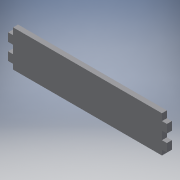
# Autodesk Inventor part: маленькое дно1
Saved by Autodesk Inventor 2019 (Build 230136000, 136)
## iProperties
Created: 2022-02-24
Part Number: маленькое дно1
Material: Типовые
Document SubType Name: Modeling
Designer: korsh
Density: 1 g/cm^3
Appearance: По умолчанию
Author: korsh
Autodesk Inventor part; units mm, degrees
ref_plane "YZ Plane" through (0, 0, 0) normal (1, 0, 0) x (0, 1, 0)
ref_plane "XZ Plane" through (0, 0, 0) normal (0, 1, 0) x (-1, 0, 0)
ref_plane "XY Plane" through (0, 0, 0) normal (0, 0, 1) x (1, 0, 0)
sketch "Эскиз1" plane through (0, 0, 0) normal (0, 0, 1) x (1, 0, 0)
  line L0 (0, 0) -> (0, -10) projected
  line L1 (0, 0) -> (-6, 0) projected
  line L2 (-6, -10) -> (-6, 0) projected
  line L3 (0, -10) -> (-6, -10) projected
  line L4 (0, -20) -> (0, -30) projected
  line L5 (0, -20) -> (-6, -20) projected
  line L6 (-6, -30) -> (-6, -20) projected
  line L7 (0, -30) -> (-6, -30) projected
  line L8 (0, -30) -> (0, -36.0265) projected
  line L9 (0, 8.1888) -> (0, 0) projected
  line L10 (186, -20) -> (186, -30) projected
  line L11 (186, -20) -> (180, -20) projected
  line L12 (180, -30) -> (180, -20) projected
  line L13 (186, -30) -> (180, -30) projected
  line L14 (186, 0) -> (186, -10) projected
  line L15 (186, 0) -> (180, 0) projected
  line L16 (180, -10) -> (180, 0) projected
  line L17 (186, -10) -> (180, -10) projected
  line L18 (180, -36.0265) -> (180, -30) projected
  line L19 (180, 0) -> (180, 8.1888) projected
  line L20 (0, 8.1888) -> (180, 8.1888)
  line L21 (180, 8.1888) -> (180, -36.0265)
  line L22 (180, -36.0265) -> (0, -36.0265)
  line L23 (0, -36.0265) -> (0, 8.1888)
  constraints: 8 end point, 2 parallel, 1 horizontal, 1 perpendicular
extrude "Выдавливание1" add sketch "Эскиз1" along normal blind 6
